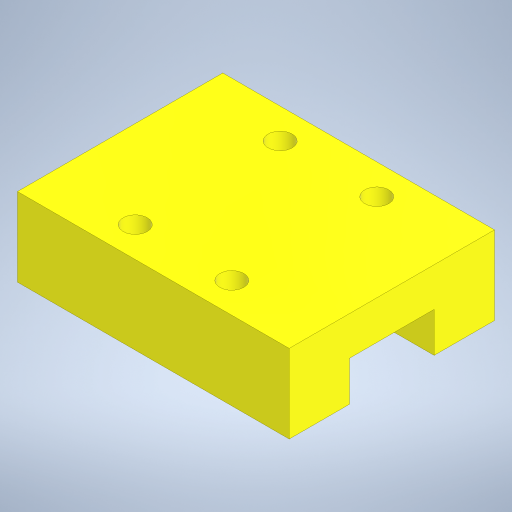
# Autodesk Inventor part: MGN7C_slider
Saved by Autodesk Inventor 2024 (Build 280153000, 153)
## iProperties
Created: 2023-08-26
Part Number: MGN7C_slider
Material: ABS Plastic
Document SubType Name: Modeling
Designer: l1534
Density: 1.06 g/cm^3
Appearance: Smooth - Yellow
Author: l1534
Autodesk Inventor part; units mm, degrees
ref_plane "YZ Plane" through (0, 0, 0) normal (1, 0, 0) x (0, 1, 0)
ref_plane "XZ Plane" through (0, 0, 0) normal (0, 1, 0) x (-1, 0, 0)
ref_plane "XY Plane" through (0, 0, 0) normal (0, 0, 1) x (1, 0, 0)
sketch "Sketch1" plane through (0, 0, 0) normal (1, 0, 0) x (0, 1, 0)
  line L0 (5.7363, 8.6903) -> (-0.7637, 8.6903)
  line L1 (-0.7637, 8.6903) -> (-0.7637, 3.6903)
  line L2 (-0.7637, 3.6903) -> (2.5363, 3.6903)
  line L3 (2.5363, 3.6903) -> (2.5363, -3.3097)
  line L4 (2.5363, -3.3097) -> (-0.7637, -3.3097)
  line L5 (-0.7637, -3.3097) -> (-0.7637, -8.3097)
  line L6 (-0.7637, -8.3097) -> (5.7363, -8.3097)
  line L7 (5.7363, -8.3097) -> (5.7363, 8.6903)
  point P0 (0, 0)
  dimension "d0" = 17
  dimension "d1" = 3.3
  dimension "d2" = 6.5
  dimension "d3" = 5
  dimension "d4" = 7
  constraints: 16 end point, 6 perpendicular, 2 point on line, 1 horizontal
  measures "d0" distance of L6.end L0.start
  measures "d1" distance of L3.end L4.end
  measures "d2" distance of L5.end L6.end
  measures "d3" distance of L4.end L5.end
  measures "d4" distance of L2.end L3.end
extrude "Extrusion1" add sketch "Sketch1" along normal blind 22.5
sketch "Sketch2" plane through (0, 5.7363, 8.6903) normal (0, 1, 0) x (1, 0, 0)
  circle A0 centre (7.25, 2.5) radius 1
  circle A1 centre (15.25, 2.5) radius 1
  circle A2 centre (15.25, 14.5) radius 1
  circle A3 centre (7.25, 14.5) radius 1
  line L0 (0, 0) -> (22.5, 0) projected
  line L1 (22.5, 17) -> (22.5, 0) projected
  line L2 (0, 17) -> (0, 0) projected
  point P0 (0, 8.6903)
  dimension "d7" = 8
  dimension "d8" = 2
  dimension "d10" = 2
  dimension "d12" = 2
  dimension "d13" = 2
  dimension "d14" = 12
  dimension "d15" = 12
  dimension "d16" = 2.5
  dimension "d17" = 7.25
  dimension "d18" = 7.25
  dimension "d20" = 8
  dimension "d21" = 2.5
  constraints: 4 centre point
  measures "d7" distance of A1.centre A0.centre
  measures "d8" diameter of A0
  measures "d10" diameter of A3
  measures "d12" diameter of A2
  measures "d13" diameter of A1
  measures "d14" distance of A3.centre A0.centre
  measures "d15" distance of A2.centre A1.centre
  measures "d16" distance from line of L0 A1.centre
  measures "d17" distance from line of L1 A2.centre
  measures "d18" distance from line of L1 A1.centre
  measures "d20" distance of A2.centre A3.centre
  measures "d21" distance from line of L0 A0.centre
extrude "Extrusion2" cut sketch "Sketch2" against normal through all
body "Solid1"
